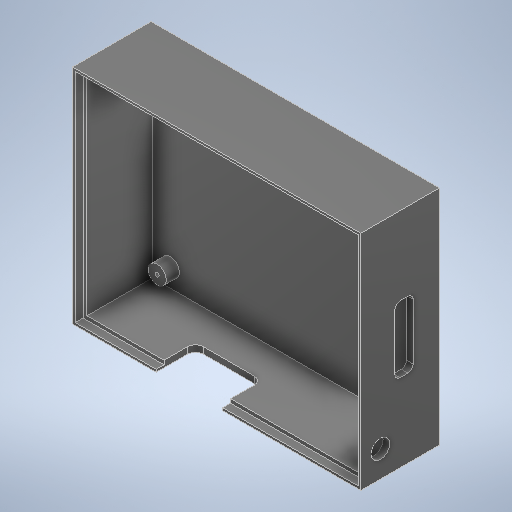
# Autodesk Inventor part: Case
Saved by Autodesk Inventor 2025 (Build 290162000, 162)
## iProperties
Created: 2024-09-04
Part Number: Case
Material: ABS plástico
Document SubType Name: Modeling
Designer: Andre
Density: 1.06 g/cm^3
Appearance: Suave - Branco
Author: Andre
Autodesk Inventor part; units mm, degrees
ref_plane "YZ Plane" through (0, 0, 0) normal (1, 0, 0) x (0, 1, 0)
ref_plane "XZ Plane" through (0, 0, 0) normal (0, 1, 0) x (-1, 0, 0)
ref_plane "XY Plane" through (0, 0, 0) normal (0, 0, 1) x (1, 0, 0)
sketch "Esboço1" plane through (0, 0, 0) normal (0, 0, 1) x (1, 0, 0)
  line L0 (-55, -42.5) -> (55, -42.5)
  line L1 (55, -42.5) -> (55, 42.5)
  line L2 (55, 42.5) -> (-55, 42.5)
  line L3 (-55, 42.5) -> (-55, -42.5)
  line L4 (-55, -42.5) -> (55, 42.5) construction
  line L5 (55, -42.5) -> (-55, 42.5) construction
  point P0 (0, 0)
  dimension "d0" = 110
  dimension "d1" = 85
  constraints: 12 end point, 2 midpoint, 2 parallel, 1 horizontal, 1 perpendicular
  measures "d0" distance of L2.end L1.end
  measures "d1" distance of L1.end L0.end
extrude "Extrusão1" add sketch "Esboço1" along normal blind 2
sketch "Esboço2" plane through (0, 0, 2) normal (0, 0, 1) x (1, 0, 0)
  line L0 (55, 42.5) -> (-55, 42.5) projected
  line L1 (55, -42.5) -> (-55, -42.5)
  line L2 (-55, -42.5) -> (-55, 42.5)
  line L3 (-55, 42.5) -> (55, 42.5)
  line L4 (55, 42.5) -> (55, -42.5)
  line L5 (55, -42.5) -> (-55, 42.5) construction
  line L6 (-55, -42.5) -> (55, 42.5) construction
  line L7 (52.5, -40) -> (-52.5, -40)
  line L8 (-52.5, -40) -> (-52.5, 40)
  line L9 (-52.5, 40) -> (52.5, 40)
  line L10 (52.5, 40) -> (52.5, -40)
  line L11 (52.5, -40) -> (-52.5, 40) construction
  line L12 (-52.5, -40) -> (52.5, 40) construction
  point P0 (0, 0)
  point P1 (55, 42.5)
  dimension "d4" = 105
  dimension "d5" = 80
  constraints: 24 end point, 4 midpoint, 4 parallel, 2 horizontal, 2 perpendicular
  measures "d4" distance of L8.end L9.end
  measures "d5" distance of L7.end L8.end
extrude "Extrusão2" add sketch "Esboço2" along normal blind 25
sketch "Esboço3" plane through (0, 0, 2) normal (0, 0, 1) x (1, 0, 0)
  line L0 (-45.72, -33.02) -> (45.72, 33.02) construction
  line L1 (45.72, -33.02) -> (-45.72, 33.02) construction
  circle A0 centre (-45.72, 33.02) radius 3.5
  circle A1 centre (45.72, 33.02) radius 3.5
  circle A2 centre (-45.72, -33.02) radius 3.5
  circle A3 centre (45.72, -33.02) radius 3.5
  circle A4 centre (-45.72, 33.02) radius 0.75
  circle A5 centre (45.72, 33.02) radius 0.75
  circle A6 centre (-45.72, -33.02) radius 0.75
  circle A7 centre (45.72, -33.02) radius 0.75
  point P0 (0, 0)
  dimension "d10" = 7
  dimension "d11" = 7
  dimension "d12" = 7
  dimension "d13" = 7
  dimension "d20" = 1.5
  dimension "d21" = 1.5
  dimension "d22" = 1.5
  dimension "d23" = 1.5
  constraints: 8 centre point, 8 coincident, 4 end point, 2 midpoint
  measures "d10" diameter of A0
  measures "d11" diameter of A1
  measures "d12" diameter of A2
  measures "d13" diameter of A3
  measures "d20" diameter of A4
  measures "d21" diameter of A5
  measures "d22" diameter of A6
  measures "d23" diameter of A7
extrude "Extrusão3" add sketch "Esboço3" along normal blind 5
sketch "Esboço4" plane through (0, 0, 27) normal (0, 0, 1) x (1, 0, 0)
  line L0 (55, -42.5) -> (-55, -42.5)
  line L1 (-55, -42.5) -> (-55, 42.5)
  line L2 (-55, 42.5) -> (55, 42.5)
  line L3 (55, 42.5) -> (55, -42.5)
  line L4 (55, -42.5) -> (-55, 42.5) construction
  line L5 (-55, -42.5) -> (55, 42.5) construction
  line L6 (54, -41.5) -> (-54, -41.5)
  line L7 (-54, -41.5) -> (-54, 41.5)
  line L8 (-54, 41.5) -> (54, 41.5)
  line L9 (54, 41.5) -> (54, -41.5)
  line L10 (54, -41.5) -> (-54, 41.5) construction
  line L11 (-54, -41.5) -> (54, 41.5) construction
  point P0 (0, 0)
  dimension "d16" = 108
  dimension "d17" = 83
  constraints: 24 end point, 4 midpoint, 4 parallel, 2 horizontal, 2 perpendicular
  measures "d16" distance of L7.end L8.end
  measures "d17" distance of L6.end L7.end
extrude "Extrusão4" add sketch "Esboço4" along normal blind 3
sketch "Esboço8" plane through (-55, -42.5, 0) normal (0, -1, 0) x (1, 0, 0)
  line L0 (31.9, 15) -> (57.3, 15)
  line L1 (57.3, 15) -> (57.3, 30)
  line L2 (57.3, 30) -> (31.9, 30)
  line L3 (31.9, 30) -> (31.9, 15)
  line L4 (0, 30) -> (110, 30) projected
  line L5 (0, 0) -> (0, 30) projected
  point P0 (53.5, 0)
  dimension "d55" = 25.4
  dimension "d56" = 15
  dimension "d57" = 31.9
  constraints: 8 end point, 2 collinear, 2 parallel, 1 horizontal, 1 perpendicular
  measures "d55" distance of L2.end L1.end
  measures "d56" distance of L1.end L0.end
  measures "d57" distance between parallel lines of L5 L3
extrude "Extrusão5" cut sketch "Esboço8" against normal blind 3
fillet "Arredondamento5" radius 3 2 edges at (-23.1, -41.25, 15) (2.3, -41.25, 15)
sketch "Esboço11" plane through (55, -42.5, 0) normal (1, 0, 0) x (0, 0, -1)
  line L0 (-30, 0) -> (-30, 85) projected
  line L1 (0, 0) -> (-30, 0) projected
  point P0 (0, 42.5)
  point P1 (-22.5, 10)
  dimension "d66" = 7.5
  dimension "d67" = 10
  measures "d66" distance from line of L0 point (-22.5, 10)
  measures "d67" distance from line of L1 point (-22.5, 10)
hole "Furo1" at (55, -32.5, 22.5) direction (-1, 0, 0) diameter 7 depth 2.5
sketch "Esboço12" plane through (55, -42.5, 0) normal (1, 0, 0) x (0, 0, -1)
  line L0 (-17, 29.8) -> (-10, 29.8)
  line L1 (-10, 29.8) -> (-10, 55.2)
  line L2 (-10, 55.2) -> (-17, 55.2)
  line L3 (-17, 55.2) -> (-17, 29.8)
  line L4 (0, 0) -> (-30, 0) projected
  line L5 (0, 0) -> (0, 85) projected
  point P0 (0, 42.5)
  point P1 (-13.5, 29.8)
  point P2 (-10, 42.5)
  point P3 (0, 42.5)
  dimension "d68" = 7
  dimension "d69" = 25.4
  dimension "d71" = 10
  constraints: 8 end point, 3 midpoint, 2 parallel, 1 horizontal, 1 horizontal alignment, 1 perpendicular
  measures "d68" distance of L2.end L1.end
  measures "d69" distance of L1.end L0.end
  measures "d71" distance between parallel lines of L5 L1
extrude "Extrusão8" cut sketch "Esboço12" against normal blind 3
fillet "Arredondamento6" radius 2 4 edges at (53.75, -12.7, 10) (53.75, -12.7, 17) (53.75, 12.7, 17) (53.75, 12.7, 10)
